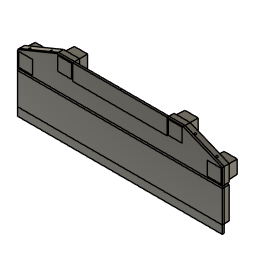
Lid Assembly v15 (Autodesk Fusion 360 archive; units mm, degrees)
design "Lid Brackets"
Autodesk Fusion 360 part; units mm, degrees
note: some values were not read from the file. Chosen so that the rebuilt part matches the saved one: that a step has no effect. Set by a fixed rule: which sketch regions a step uses.
sketch "Sketch1" plane through (0, 0, 0) normal (0, 1, 0) x (1, 0, 0)
  line L0 (0, 0) -> (325, 0)
  line L1 (325, 0) -> (325, -50)
  line L2 (325, -50) -> (0, -50)
  line L3 (0, -50) -> (0, 0)
  line L4 (0, 0) -> (325.0012, 0)
  line L5 (325.0012, 0) -> (325.0012, 13)
  line L6 (325.0012, 13) -> (0, 13)
  line L7 (0, 13) -> (0, 0)
  line L8 (162.5006, -104.25) -> (162.5006, 13)
  line L9 (323.2506, -77) -> (323.2506, -55)
  line L10 (301.2506, -77) -> (323.2506, -77)
  line L11 (301.2506, -55) -> (301.2506, -77)
  line L12 (323.2506, -55) -> (301.2506, -55)
  line L13 (299.5039, -53.25) -> (299.5061, -78.75)
  line L14 (0, -53.25) -> (325, -53.25)
  line L15 (23.7506, -55) -> (23.7506, -77)
  line L16 (23.7506, -77) -> (1.7506, -77)
  line L17 (1.7506, -77) -> (1.7506, -55)
  line L18 (1.7506, -55) -> (23.7506, -55)
  line L19 (25.4972, -53.25) -> (25.4951, -78.75)
  line L20 (325, -50) -> (325, -53.25)
  line L21 (325, -53.25) -> (325, -78.75)
  line L22 (0, -50) -> (0, -53.25)
  line L23 (0, -53.25) -> (0, -78.75)
  line L24 (0, -78.75) -> (25.5, -78.75)
  line L25 (325, -78.75) -> (0, -78.75)
  line L26 (0, -78.75) -> (62, -78.75)
  line L27 (62, -78.75) -> (87.5, -78.75)
  line L28 (87.5, -78.75) -> (87.5, -104.25)
  line L29 (87.5, -104.25) -> (62, -104.25)
  line L30 (62, -104.25) -> (62, -78.75)
  line L31 (63.75, -80.5) -> (85.75, -80.5)
  line L32 (85.75, -80.5) -> (85.75, -102.5)
  line L33 (85.75, -102.5) -> (63.75, -102.5)
  line L34 (63.75, -102.5) -> (63.75, -80.5)
  line L35 (0, -78.75) -> (62, -104.25)
  line L36 (62, -104.25) -> (162.5006, -104.25)
  line L37 (237.5012, -78.75) -> (237.5012, -104.25)
  line L38 (261.2512, -80.5) -> (239.2512, -80.5)
  line L39 (239.2512, -102.5) -> (261.2512, -102.5)
  line L40 (261.2512, -102.5) -> (261.2512, -80.5)
  line L41 (325.0012, -78.75) -> (263.0012, -104.25)
  line L42 (325.0012, -78.75) -> (263.0012, -78.75)
  line L43 (263.0012, -78.75) -> (237.5012, -78.75)
  line L44 (325.0012, -78.75) -> (299.5012, -78.75)
  line L45 (239.2512, -80.5) -> (239.2512, -102.5)
  line L46 (263.0012, -104.25) -> (263.0012, -78.75)
  line L47 (237.5012, -104.25) -> (263.0012, -104.25)
  line L48 (263.0012, -104.25) -> (162.5006, -104.25)
  dimension "d1" = 325
  dimension "d2" = 50
  dimension "d4" = 13
  dimension "d54" = 3.25
  dimension "d58" = 25.5
  dimension "d60" = 3.25
  dimension "d62" = 25.5
  dimension "d65" = 62
  dimension "d66" = 25.5
  dimension "d67" = 25.5
  dimension "d68" = 1.75
  constraint horizontal L0
  constraint vertical L1
  constraint horizontal L2
  constraint vertical L3
  constraint coincident L0.start L3.end
  constraint horizontal L4
  constraint vertical L5
  constraint horizontal L6
  constraint vertical L7
  constraint midpoint L6 L8.end
  constraint symmetric L8 L13.end L19.end
  constraint symmetric L8 L9.start L16.end
  constraint symmetric L8 L13.start L19.start
  constraint symmetric L8 L9.end L17.end
  constraint symmetric L8 L11.start L15.start
  constraint symmetric L8 L10.start L15.end
  constraint perpendicular L2 L20
  constraint perpendicular L14 L21
  constraint perpendicular L14 L22
  constraint perpendicular L14 L23
  constraint perpendicular L23 L24
  constraint perpendicular L23 L25
  constraint perpendicular L23 L26
  constraint horizontal L27
  constraint vertical L28
  constraint horizontal L29
  constraint vertical L30
  constraint symmetric L23.end L8 L41.start
  constraint symmetric L8 L36.end L48.end
  constraint symmetric L8 L24.end L44.end
  constraint symmetric L8 L26.end L42.end
  constraint symmetric L8 L27.end L37.start
  constraint symmetric L8 L28.end L37.end
  constraint symmetric L8 L29.end L41.end
  constraint symmetric L8 L31.start L38.start
  constraint symmetric L8 L31.end L38.end
  constraint symmetric L8 L32.end L39.start
  constraint symmetric L8 L33.end L39.end
  measures "d1" distance of L0.start L0.end
  measures "d2" distance of L0.start L2.end
  measures "d4" distance of L0.start L6.end
  measures "d54" distance of L2.end L14.start
  measures "d58" distance of L23.end L14.start
  measures "d60" distance of L1.end L14.end
  measures "d62" distance of L23.end L24.end
  measures "d65" distance of L23.end L26.end
  measures "d66" distance of L26.end L27.end
  measures "d67" distance of L26.end L29.end
combine "Combine1" [no effect]
extrude "Extrude13" add sketch "Sketch1" along normal blind 3 contours L0 L4 L6 L7 L8 | L0 L2 L3 L4 L8 | L0 L4 L5 L6 L8 | L0 L1 L2 L4 L8 | L2 L8 L14 L22 | L2 L8 L14 L20 | L14 L19 L23 L24 L25 L26 | L8 L13 L14 L25 L42 L43 L44 | L8 L14 L19 L24 L25 L26 L27 | L24 L25 L26 L30 L35 | L13 L14 L21 L25 L42 L44 | L8 L25 L37 L48 | L8 L25 L28 L36 | L25 L27 L28 L29 L30 L36 | L25 L41 L42 L44 L46 | L25 L37 L43 L46 L47 L48 | L9 L10 L11 L12 | L15 L16 L17 L18 | L31 L32 L33 L34 | L38 L39 L40 L45 makes body 1
extrude "Extrude14" add sketch "Sketch1" along normal blind 11 separate body contours L0 L2 L3 L4 L8 | L0 L1 L2 L4 L8 | L14 L19 L23 L24 L25 L26 | L8 L13 L14 L25 L42 L43 L44 | L8 L14 L19 L24 L25 L26 L27 | L24 L25 L26 L30 L35 | L13 L14 L21 L25 L42 L44 | L25 L27 L28 L29 L30 L36 | L25 L41 L42 L44 L46 | L25 L37 L43 L46 L47 L48 | L9 L10 L11 L12 | L15 L16 L17 L18 | L31 L32 L33 L34 | L38 L39 L40 L45 makes body 2 at (108.3333, 0, 33.3333) makes body 3 at (49.8333, 0, 78.75)
extrude "Extrude15" add sketch "Sketch1" along normal blind 26 separate body contours L9 L10 L11 L12 | L15 L16 L17 L18 | L31 L32 L33 L34 | L38 L39 L40 L45 makes body 4 at (261.2512, 8.6667, 95.1667) makes body 5 at (71.0833, 8.6667, 80.5) makes body 6 at (301.2506, 8.6667, 62.3333) makes body 7 at (23.7506, 17.3333, 62.3333)
chamfer "Chamfer3" distance 0.5 distance2 15 16 edges at (85.75, 26, 91.5) (74.75, 26, 102.5) (74.75, 26, 80.5) (63.75, 26, 91.5) (250.2512, 26, 102.5) (261.2512, 26, 91.5) (250.2512, 26, 80.5) (239.2512, 26, 91.5) (323.2506, 26, 66) (312.2506, 26, 77) (301.2506, 26, 66) (312.2506, 26, 55) (23.7506, 26, 66) (12.7506, 26, 55) (1.7506, 26, 66) (12.7506, 26, 77) measured on face at (71.0833, 26, 87.8333) measured on face at (71.0833, 26, 87.8333) measured on face at (71.0833, 26, 87.8333) measured on face at (71.0833, 26, 87.8333) measured on face at (253.9178, 26, 87.8333) measured on face at (253.9178, 26, 87.8333) measured on face at (253.9178, 26, 87.8333) measured on face at (253.9178, 26, 87.8333) measured on face at (308.5839, 26, 69.6667) measured on face at (308.5839, 26, 69.6667) measured on face at (308.5839, 26, 69.6667) measured on face at (308.5839, 26, 69.6667) measured on face at (16.4173, 26, 69.6667) measured on face at (16.4173, 26, 69.6667) measured on face at (16.4173, 26, 69.6667) measured on face at (16.4173, 26, 69.6667) on bodies 4 5 6 7
sketch "Sketch2" plane through (74.7257, 0, 181.6859) normal (0.380375, 0, 0.924832) x (0, 1, 0)
  line L0 (0, -203.578) -> (0, -270.6171)
  line L1 (0, -270.6171) -> (11, -270.6171)
  line L2 (11, -270.6171) -> (11, -203.578)
  line L3 (11, -203.578) -> (0, -203.578)
  line L4 (5.5, -203.578) -> (5.5, -270.6171)
  circle A0 centre (5.5, -218.578) radius 1.5
  line L5 (11, -237.0976) -> (0, -237.0976)
  circle A1 centre (5.5, -255.6171) radius 1.5
  dimension "d79" = 3
  dimension "d80" = 15
  constraint midpoint L3 L4.start
  constraint midpoint L1 L4.end
  constraint coincident L4 A0.centre
  constraint midpoint L2 L5.start
  constraint midpoint L0 L5.end
  constraint symmetric A0 L5 A1
  measures "d79" diameter of A0
  measures "d80" distance of L4.start A0.centre
extrude "Extrude17" cut sketch "Sketch2" against normal blind 20 contours L4 A0 | L4 A0 | L4 A1 | L4 A1 bodies 3 6
ref_plane "WorkPlane1" through (162.5006, 3, 104.25) normal (-1, 0, 0) x (0, -1, 0)
mirror "Mirror1" about plane through (162.5006, 3, 104.25) normal (-1, 0, 0) of "Extrude17"
sketch "Sketch3" plane through (0, 0, 78.75) normal (0, 0, 1) x (-1, 0, 0)
  line L0 (-87.5, 0) -> (-237.5012, 0)
  line L1 (-237.5012, 0) -> (-237.5012, -11)
  line L2 (-237.5012, -11) -> (-87.5, -11)
  line L3 (-87.5, -11) -> (-87.5, 0)
  line L4 (-87.5, -5.5) -> (-237.5012, -5.5)
  circle A0 centre (-112.5, -5.5) radius 1.5
  line L5 (-162.5006, -5.5) -> (-162.5006, 0)
  circle A1 centre (-212.5012, -5.5) radius 1.5
  dimension "d85" = 3
  dimension "d86" = 25
  constraint midpoint L3 L4.start
  constraint midpoint L1 L4.end
  constraint coincident L4 A0.centre
  constraint midpoint L4 L5.start
  constraint midpoint L0 L5.end
  constraint symmetric A0 L5 A1
  measures "d85" diameter of A0
  measures "d86" distance of L4.start A0.centre
extrude "Extrude18" cut sketch "Sketch3" against normal blind 50 contours L4 A0 | L4 A0 | L4 A1 | L4 A1 bodies 2 3
combine "Combine2" [no effect]
combine "Combine3" [no effect]
